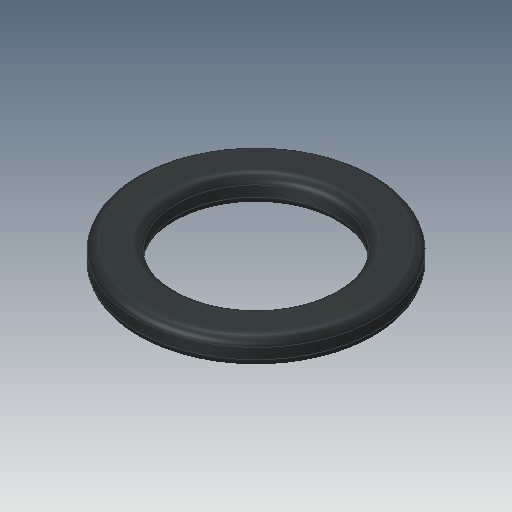
# Autodesk Inventor part: SimLing
Saved by Autodesk Inventor 2019.4 (Build 234330000, 330)
## iProperties
Created: 2019-06-15
Part Number: SimLing
Material: 鉄、ねずみ鋳鉄 ASTM A-48 グレード 50
Document SubType Name: Modeling
Designer: AzLIer
Density: 7.3953 g/cm^3
Appearance: 鉄 ねずみ鋳鉄
Mass: 0.24791 g
Surface Area: 1.05674 cm^2
Volume: 0.0335226 cm^3
Author: AzLIer
Autodesk Inventor part; units mm, degrees
ref_plane "YZ Plane" through (0, 0, 0) normal (1, 0, 0) x (0, 1, 0)
ref_plane "XZ Plane" through (0, 0, 0) normal (0, 1, 0) x (-1, 0, 0)
ref_plane "XY Plane" through (0, 0, 0) normal (0, 0, 1) x (1, 0, 0)
sketch "スケッチ1" plane through (0, 0, 0) normal (0, 1, 0) x (-1, 0, 0)
  circle A0 centre (0, 0) radius 3
  circle A1 centre (0, 0) radius 4.5
  dimension "d0" = 6
  dimension "d1" = 9
  constraints: 2 centre point, 2 coincident
  measures "d0" diameter of A0
  measures "d1" diameter of A1
extrude "押し出し1" add sketch "スケッチ1" along normal blind 1
fillet "フィレット1" radius 0.3 4 edges at (3, 1, 0) (3, 0, 0) (4.5, 1, 0) (4.5, 0, 0)
